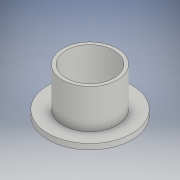
# Autodesk Inventor part: Шайба_Уплотнитель
Saved by Autodesk Inventor 2017 (Build 210142000, 142)
## iProperties
Part Number: Шайба_Уплотнитель
Material: Типовые
Document SubType Name: Modeling
Designer: yulia_000
Density: 1 g/cm^3
Appearance: По умолчанию
Author: yulia_000
Autodesk Inventor part; units mm, degrees
ref_plane "YZ Plane" through (0, 0, 0) normal (1, 0, 0) x (0, 1, 0)
ref_plane "XZ Plane" through (0, 0, 0) normal (0, 1, 0) x (-1, 0, 0)
ref_plane "XY Plane" through (0, 0, 0) normal (0, 0, 1) x (1, 0, 0)
sketch "Эскиз1" plane through (0, 0, 0) normal (0, 1, 0) x (-1, 0, 0)
  circle A0 centre (0, 0) radius 7.5
  dimension "d0" = 15
  constraints: 1 centre point, 1 coincident
  measures "d0" diameter of A0
extrude "Выдавливание1" add sketch "Эскиз1" along normal blind 1
sketch "Эскиз2" plane through (0, 1, 0) normal (0, 1, 0) x (1, 0, 0)
  circle A0 centre (0, 0) radius 7.5 projected
  circle A1 centre (0, 0) radius 4.9
  dimension "d3" = 9.8
  constraints: 1 centre point, 1 coincident
  measures "d3" diameter of A1
extrude "Выдавливание2" add sketch "Эскиз2" along normal blind 7 contours A1
sketch "Эскиз4" plane through (0, 8, 0) normal (0, 1, 0) x (1, 0, 0)
  circle A0 centre (0, 0) radius 4.9 projected
  circle A1 centre (0, 0) radius 4.3
  dimension "d9" = 8.6
  constraints: 1 centre point, 1 coincident
  measures "d9" diameter of A1
extrude "Выдавливание4" cut sketch "Эскиз4" against normal through all contours A1
